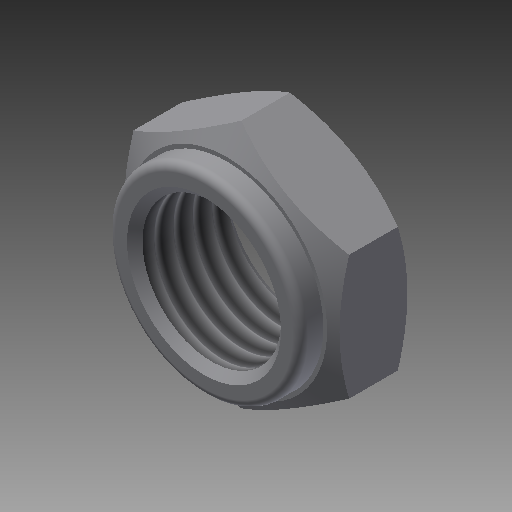
# Autodesk Inventor part: Dado 14
Saved by Autodesk Inventor 2019 (Build 230136000, 136)
## iProperties
Created: 2011-09-22
Part Number: Dado 14
Document SubType Name: Modeling
Designer: Stefano
Density: 1 g/cm^3
Material: 一般
Appearance: 既定
Author: Stefano
Autodesk Inventor part; units mm, degrees
ref_plane "YZ Plane" through (0, 0, 0) normal (1, 0, 0) x (0, 1, 0)
ref_plane "XZ Plane" through (0, 0, 0) normal (0, 1, 0) x (-1, 0, 0)
ref_plane "XY Plane" through (0, 0, 0) normal (0, 0, 1) x (1, 0, 0)
sketch "Schizzo1" plane through (0, 0, 0) normal (0, 0, 1) x (1, 0, 0)
  line L0 (0, 8.0829) -> (7, 4.0415)
  line L1 (7, 4.0415) -> (7, -4.0415)
  line L2 (7, -4.0415) -> (0, -8.0829)
  line L3 (0, -8.0829) -> (-7, -4.0415)
  line L4 (-7, -4.0415) -> (-7, 4.0415)
  line L5 (-7, 4.0415) -> (0, 8.0829)
  point P0 (0, 0)
  point P1 (0, 0)
  dimension "d0" = 14
  constraints: 12 end point, 1 coincident, 13 other
  measures "d0" distance between parallel lines of L1 L4
extrude "Estrusione1" add sketch "Schizzo1" along normal blind 5
sketch "Schizzo2" plane through (0, 0, 5) normal (0, 0, 1) x (1, 0, 0)
  circle A0 centre (0, 0) radius 6.25
  dimension "d5" = 12.5
  constraints: 1 centre point, 1 coincident
  measures "d5" diameter of A0
extrude "Estrusione2" add sketch "Schizzo2" along normal blind 1.5
sketch "Schizzo3" plane through (0, 0, 0) normal (1, 0, 0) x (0, 1, 0)
  line L0 (8.0829, 5) -> (4.0415, 5) projected
  line L1 (4.0415, 0) -> (4.0415, 5) projected
  line L2 (8.0829, 0) -> (4.0415, 0) projected
  line L3 (8.0829, 0) -> (8.0829, 5) projected
  line L4 (6.4929, 0) -> (8.0829, 0.918)
  line L5 (0, -0.8) -> (0, 4.8) projected
  line L6 (6.4929, 5) -> (8.0829, 4.082)
  line L7 (6.4929, 5) -> (8.0829, 5)
  line L8 (8.0829, 4.082) -> (8.0829, 5)
  point P0 (0, 0)
  dimension "d6" = 30
  constraints: 8 end point, 2 collinear, 2 point on line
  measures "d6" angle of L4 L2
ref_plane "Piano di lavoro1" through (0, 0, 2) normal (0, 0, -1) x (-1, 0, 0)
sketch "Schizzo4" plane through (0, 0, 6.5) normal (0, 0, 1) x (1, 0, 0)
  circle A0 centre (0, 0) radius 6.25 projected
hole "Foro1" at (0, 0, 6.5) direction (0, 0, -1) diameter 9 end through all
thread "Filettatura1" size "M9x1.25" class "6H" standard "ANSI Metric M Profile" full length
chamfer "Smusso1" distance 0.5 angle 45 2 edges at (0, 4.5, 6.5) (0, 4.5, 0)
revolve "Rivoluzione2" cut sketch "Schizzo3" angle 360 about axis through (0, 0, -10) along (0, 0, 1) contours L3 L6 L0 | L3 L2 L4
fillet "Raccordo1" radius 0.5 1 edges at (-6.25, 0, 6.5)
